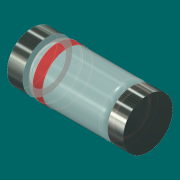
# Autodesk Inventor part: sod-80
Saved by Autodesk Inventor 2016 (Build 200138000, 138)
## iProperties
Created: 2015-11-05
Part Number: sod-80
Material: Glass
Document SubType Name: Modeling
Designer: Sawaiz
Density: 2.18 g/cm^3
Appearance: Clear
Author: Sawaiz
Autodesk Inventor part; units mm, degrees
ref_plane "YZ Plane" through (0, 0, 0) normal (1, 0, 0) x (0, 1, 0)
ref_plane "XZ Plane" through (0, 0, 0) normal (0, 1, 0) x (-1, 0, 0)
ref_plane "XY Plane" through (0, 0, 0) normal (0, 0, 1) x (1, 0, 0)
sketch "Sketch1" plane through (0, 0, 0) normal (0, 0, 1) x (1, 0, 0)
  line L0 (-0.75, -1.75) -> (0.75, -1.75)
  line L1 (0.75, -1.75) -> (0.75, 1.75)
  line L2 (0.75, 1.75) -> (-0.75, 1.75)
  line L3 (-0.75, 1.75) -> (-0.75, -1.75)
  line L4 (-0.75, -1.75) -> (0.75, 1.75) construction
  line L5 (0.75, -1.75) -> (-0.75, 1.75) construction
  line L6 (-0.75, -1.28) -> (-0.55, -1.28)
  line L7 (-0.55, -1.28) -> (-0.55, -1.23)
  line L8 (-0.55, -1.23) -> (-0.75, -1.23)
  line L9 (-0.75, -1.23) -> (-0.75, -1.28)
  line L10 (-0.75, 1.23) -> (-0.55, 1.23)
  line L11 (-0.55, 1.23) -> (-0.55, 1.28)
  line L12 (-0.55, 1.28) -> (-0.75, 1.28)
  line L13 (-0.75, 1.28) -> (-0.75, 1.23)
  line L14 (0, -1.75) -> (0, 1.75)
  line L15 (-0.75, -0.98) -> (-0.76, -0.98)
  line L16 (-0.76, -0.98) -> (-0.76, -0.68)
  line L17 (-0.76, -0.68) -> (-0.75, -0.68)
  line L18 (-0.75, -0.68) -> (-0.75, -0.98)
  point P0 (0, 0)
  dimension "d0" = 1.5
  dimension "d1" = 3.5
  dimension "d2" = 0.47
  dimension "d3" = 0.05
  dimension "d4" = 0.47
  dimension "d5" = 0.05
  dimension "d6" = 0.2
  dimension "d9" = 0.01
  dimension "d10" = 0.25
  dimension "d11" = 0.3
  constraints: 38 end point, 8 parallel, 4 horizontal, 4 midpoint, 4 perpendicular, 4 point on line
  measures "d0" distance of L2.end L1.end
  measures "d1" distance of L1.end L0.end
  measures "d2" distance between parallel lines of L0 L6
  measures "d3" distance between parallel lines of L8 L6
  measures "d4" distance between parallel lines of L2 L12
  measures "d5" distance between parallel lines of L12 L10
  measures "d6" distance between parallel lines of L3 L11
  measures "d9" distance between parallel lines of L18 L16
  measures "d10" distance between parallel lines of L8 L15
  measures "d11" distance between parallel lines of L15 L17
revolve "Revolution1" add sketch "Sketch1" angle 360 about axis through (0, -1.75, 0) along (0, 1, 0) contours L3 L6 L7 L8 L10 L11 L12 L2 L14 L0 | L15 L16 L17 L3
fillet "Fillet1" radius 0.2 2 edges at (0.75, -1.23, 0) (0.75, 1.23, 0)
body "Solid1"
